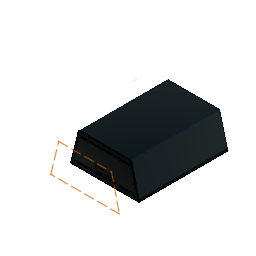
Assembly 4 v6 (Autodesk Fusion 360 archive; units mm, degrees)
design "Container_LeftBack"
Autodesk Fusion 360 part; units mm, degrees
sketch "Sketch1" plane through (0, 0, 0) normal (0, 1, 0) x (1, 0, 0)
  line L0 (-40, 14) -> (125, 14)
  line L1 (-20.5, -60) -> (105.5, -60)
  line L2 (-20.5, -60) -> (-40, 14)
  line L3 (105.5, -60) -> (125, 14)
  line L4 (-45.1906, 18) -> (130.1906, 18)
  line L5 (108.5825, -64) -> (130.1906, 18)
  line L6 (-23.5825, -64) -> (108.5825, -64)
  line L7 (-23.5825, -64) -> (-45.1906, 18)
  dimension "d6" = 4
  constraint horizontal L0
  constraint parallel L0 L1
extrude "Extrude1" add sketch "Sketch1" along normal blind 228
sketch "Sketch2" plane through (0, 0, 0) normal (0, 1, 0) x (1, 0, 0)
  line L0 (-45.3287, 17.7134) -> (130, 17.7134)
  line L1 (-25, -65) -> (110, -65)
  line L2 (110, -65) -> (130, 17.7134)
  line L3 (-25, -65) -> (-45.3287, 17.7134)
  constraint horizontal L0
  constraint horizontal L1
extrude "Extrude2" add sketch "Sketch2" along normal blind 1
sketch "Sketch3" plane through (0, 0, 0) normal (0, 1, 0) x (1, 0, 0)
  line L0 (20, 0) -> (65, 0)
  line L1 (65, 0) -> (65, -8.5)
  line L2 (65, -8.5) -> (20, -8.5)
  line L3 (20, -8.5) -> (20, 0)
  dimension "d12" = 8.5
  constraint horizontal L0
  constraint vertical L1
  constraint horizontal L2
  constraint vertical L3
  measures "d12" distance of L0.start L2.end
extrude "Extrude3" cut sketch "Sketch3" along normal blind 5
sketch "Sketch4" plane through (0, 0, 0) normal (0, 1, 0) x (1, 0, 0)
sketch "Sketch5" plane through (0, 0, 64) normal (0, 0, 1) x (-1, 0, 0)
  line L0 (23.5825, -1) -> (-108.5825, -1)
  line L1 (-108.5825, -1) -> (-108.5825, -228)
  line L2 (-108.5825, -228) -> (23.5825, -228)
  line L3 (23.5825, -228) -> (23.5825, -1)
sketch "Sketch6" plane through (0, 0, 0) normal (0, 1, 0) x (1, 0, 0)
split_face "SplitFace1" 2 faces at (20.4725, 76.6667, 64) (122.4972, 152.3333, 11.1953) by plane through (0, 0, 0) normal (0, -1, 0)
sketch "Sketch7" plane through (0, 0, 0) normal (0, 1, 0) x (1, 0, 0)
  line L0 (-25, -65, -50) -> (110, -65, -50) construction
  line L1 (110, -65, -50) -> (130.0131, 17.8851, -50) construction
  line L2 (130.0131, 17.8851, -50) -> (-45.0122, 17.8851, -50) construction
  line L3 (-45.0122, 17.8851, -50) -> (-25, -65, -50) construction
sketch "Sketch8" plane through (117.302, 0, 30.9107) normal (0.96699, 0, 0.254815) x (0, 1, 0)
  line L0 (1, -44.8037) -> (228, -44.8037)
  line L1 (228, -44.8037) -> (228, 34.2189)
  line L2 (228, 34.2189) -> (1, 34.2189)
  line L3 (1, 34.2189) -> (1, -44.8037)
sketch "Sketch9" plane through (0, 0, 0) normal (1, 0, 0) x (0, 1, 0)
sketch "Sketch10" plane through (0, 1, 0) normal (0, 1, 0) x (-1, 0, 0)
  line L0 (-20, 8.5) -> (-20, 0)
  line L1 (-20, 0) -> (-65, 0)
  line L2 (-65, 0) -> (-65, 8.5)
  line L3 (-65, 8.5) -> (-20, 8.5)
  line L4 (-105.5, 60) -> (-125, -14)
  line L5 (-125, -14) -> (40, -14)
  line L6 (40, -14) -> (20.5, 60)
  line L7 (20.5, 60) -> (-105.5, 60)
sketch "Sketch11" plane through (0, 1, 0) normal (0, 1, 0) x (-1, 0, 0)
  line L0 (-110, 55) -> (26.2971, 55)
  line L1 (26.2971, 55) -> (26.2971, 51.5)
  line L2 (26.2971, 51.5) -> (-110, 51.5)
  line L3 (-110, 51.5) -> (-110, 55)
  dimension "d16" = 3.5
  constraint horizontal L0
  constraint vertical L1
  constraint horizontal L2
  constraint vertical L3
  measures "d16" distance of L0.start L2.end
extrude "Extrude4" add sketch "Sketch11" along normal blind 227
sketch "Sketch12" plane through (0, 1, 0) normal (0, 1, 0) x (-1, 0, 0)
  line L0 (-124.605, -9) -> (40, -9)
  line L1 (40, -9) -> (40, -5.5)
  line L2 (40, -5.5) -> (-124.605, -5.5)
  line L3 (-124.605, -5.5) -> (-124.605, -9)
  dimension "d19" = 3.5
  constraint horizontal L0
  constraint vertical L1
  constraint horizontal L2
  constraint vertical L3
  measures "d19" distance of L0.start L2.end
extrude "Extrude5" add sketch "Sketch12" along normal blind 227
sketch "Sketch13" plane through (-152.3278, -0.2738, -0.1145) normal (-0.999998, -0.001797, -0.000752) x (0.001797, -0.999998, 0)
  line L0 (-277.193, -23.2673) -> (-277.1579, -25.267)
  line L1 (-277.1579, -25.267) -> (-275.1582, -25.2318)
  line L2 (-275.1582, -25.2318) -> (-262.1602, -25.0033)
  line L3 (-262.1602, -25.0033) -> (-262.1953, -23.0037)
  line L4 (-262.1953, -23.0037) -> (-277.193, -23.2673)
sketch "Sketch14" plane through (0, 228, 0) normal (0, 1, 0) x (-1, 0, 0)
  line L0 (-122.7601, -5.5) -> (-107.7399, 51.5)
  line L1 (-107.7399, 51.5) -> (22.7399, 51.5)
  line L2 (22.7399, 51.5) -> (37.7601, -5.5)
  line L3 (37.7601, -5.5) -> (-122.7601, -5.5)
  line L4 (-123.6824, -9) -> (38.6824, -9)
  line L5 (38.6824, -9) -> (40, -14)
  line L6 (40, -14) -> (-125, -14)
  line L7 (-125, -14) -> (-123.6824, -9)
  line L8 (-106.8176, 55) -> (-105.5, 60)
  line L9 (-105.5, 60) -> (20.5, 60)
  line L10 (20.5, 60) -> (21.8176, 55)
  line L11 (21.8176, 55) -> (-106.8176, 55)
  line L12 (25.9541, 55) -> (23.5825, 64)
  line L13 (23.5825, 64) -> (-108.5825, 64)
  line L14 (-108.5825, 64) -> (-128.7186, -12.414)
  line L15 (-128.7186, -12.414) -> (-130.1906, -18)
  line L16 (-130.1906, -18) -> (45.1906, -18)
  line L17 (45.1906, -18) -> (26.2971, 53.6986)
  line L18 (26.2971, 53.6986) -> (26.2971, 55)
  line L19 (26.2971, 55) -> (25.9541, 55)
  line L20 (20.5, 60) -> (26.2487, 60)
  line L21 (26.2487, 60) -> (27.5, 55)
  line L22 (27.5, 55) -> (21.8176, 55)
  line L23 (20.5, 60) -> (21.8176, 55)
  constraint coincident L9.end L10.start
  constraint parallel L9 L20
  constraint coincident L10.end L11.start
extrude "Extrude6" cut sketch "Sketch14" against normal blind 16 contours L10 L12 L20 L22 L23 | L12 L19 L20 L21 L22
sketch "Sketch15" plane through (0, 228, 0) normal (0, 1, 0) x (-1, 0, 0)
  line L0 (25.9541, 55) -> (21.8176, 55)
  line L1 (21.8176, 55) -> (-106.8176, 55)
  line L2 (-106.8176, 55) -> (-105.5, 60)
  line L3 (-105.5, 60) -> (24.6365, 60)
  line L4 (24.6365, 60) -> (23.5825, 64)
  line L5 (23.5825, 64) -> (-108.5825, 64)
  line L6 (-108.5825, 64) -> (-128.7186, -12.414)
  line L7 (-128.7186, -12.414) -> (-130.1906, -18)
  line L8 (-130.1906, -18) -> (45.1906, -18)
  line L9 (45.1906, -18) -> (26.2971, 53.6986)
  line L10 (26.2971, 53.6986) -> (26.2971, 55)
  line L11 (26.2971, 55) -> (25.9541, 55)
  line L12 (-122.7601, -5.5) -> (-107.7399, 51.5)
  line L13 (-107.7399, 51.5) -> (22.7399, 51.5)
  line L14 (22.7399, 51.5) -> (37.7601, -5.5)
  line L15 (37.7601, -5.5) -> (-122.7601, -5.5)
  line L16 (-123.6824, -9) -> (38.6824, -9)
  line L17 (38.6824, -9) -> (40, -14)
  line L18 (40, -14) -> (-125, -14)
  line L19 (-125, -14) -> (-123.6824, -9)
  line L20 (38.6824, -9) -> (43.5, -9)
  line L21 (43.5, -9) -> (44.5, -14)
  line L22 (44.5, -14) -> (40, -14)
  line L23 (38.6824, -9) -> (40, -14)
  dimension "d25" = 0
  constraint coincident L16.end L17.start
  constraint parallel L16 L20
  constraint coincident L17.end L18.start
extrude "Extrude7" cut sketch "Sketch15" against normal blind 16 contours L9 L20 L21 L22 | L9 L17 L20 L22 L23

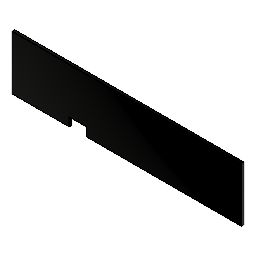
design "LC_SFPB: Left Side (Front to Back"
Autodesk Fusion 360 part; units mm, degrees
sketch "Sketch1" plane through (0, 0, 0) normal (0, 1, 0) x (1, 0, 0)
  line L0 (-110, -30) -> (290, -30)
  line L1 (290, -30) -> (290, 65)
  line L2 (290, 65) -> (-110, 65)
  line L3 (-110, 65) -> (-110, -30)
  line L4 (290, 65) -> (20, 65)
  line L5 (20, 65) -> (20, 50)
  line L6 (20, 50) -> (-10, 50)
  line L7 (-10, 50) -> (-10, 65)
  constraint horizontal L0
  constraint perpendicular L0 L1
  constraint perpendicular L1 L2
  constraint perpendicular L0 L3
  constraint coincident L2 L4.end
  constraint perpendicular L2 L5
  constraint perpendicular L5 L6
  constraint coincident L2 L7.end
  constraint perpendicular L2 L7
extrude "Extrude1" add sketch "Sketch1" along normal blind 5 contours L0 L1 L2 L3 L4 L5 L6 L7
sketch "Sketch2" plane through (0, 0, 0) normal (0, 1, 0) x (1, 0, 0)

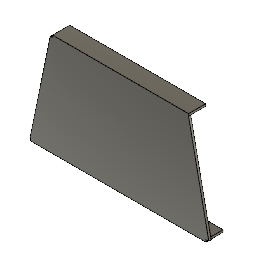
design "Door (Height needs adjustment maybe)"
Autodesk Fusion 360 part; units mm, degrees
sketch "Sketch1" plane through (0, 0, 0) normal (0, 1, 0) x (1, 0, 0)
  line L0 (-30, -40) -> (90, -40)
  line L1 (90, 45) -> (-30, 45)
  line L2 (-30, 45) -> (-47.5, 45)
  line L3 (90, 45) -> (107.5, 45)
  line L4 (-47.5, 45) -> (-30, -40)
  line L5 (107.5, 45) -> (90, -40)
  constraint horizontal L0
extrude "Extrude1" add sketch "Sketch1" along normal blind 2
sketch "Sketch2" plane through (0, 0, 0) normal (1, 0, 0) x (0, 1, 0)
  line L0 (0, 40) -> (15, 40)
  line L1 (15, 40) -> (15, 42)
  line L2 (15, 42) -> (0, 42)
  line L3 (0, 42) -> (0, 40)
  line L4 (0, -45) -> (0, -47)
  line L5 (0, -47) -> (15, -47)
  line L6 (15, -47) -> (15, -45)
  line L7 (15, -45) -> (0, -45)
  constraint horizontal L0
  constraint perpendicular L0 L1
  constraint perpendicular L1 L2
  constraint perpendicular L0 L3
  constraint vertical L4
  constraint perpendicular L4 L5
  constraint perpendicular L5 L6
  constraint perpendicular L4 L7
extrude "Extrude2" add sketch "Sketch2" along normal blind 105 and the other way blind 47 contours L4 L5 L6 L7
sketch "Sketch3" plane through (0, 0, 0) normal (1, 0, 0) x (0, 1, 0)
  line L0 (0, 40) -> (15, 40)
  line L1 (15, 40) -> (15, 42)
  line L2 (15, 42) -> (0, 42)
  line L3 (0, 42) -> (0, 40)
  constraint horizontal L0
  constraint perpendicular L0 L1
  constraint perpendicular L1 L2
  constraint perpendicular L0 L3
extrude "Extrude3" add sketch "Sketch3" along normal blind 90 and the other way blind 28

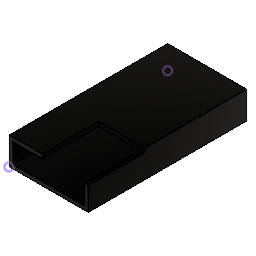
design "Left Pavement"
Autodesk Fusion 360 part; units mm, degrees
sketch "Sketch1" plane through (0, 0, 0) normal (0, 1, 0) x (1, 0, 0)
  line L0 (-30, 0) -> (70, 0)
  line L1 (70, 0) -> (70, -35)
  line L2 (70, -35) -> (-30, -35)
  line L3 (-30, -35) -> (-30, 0)
  line L4 (-25, -5) -> (65, -5)
  line L5 (65, -5) -> (65, -30)
  line L6 (65, -30) -> (-25, -30)
  line L7 (-25, -30) -> (-25, -5)
  dimension "d1" = 35
  dimension "d2" = 5
  constraint horizontal L0
  constraint perpendicular L0 L1
  constraint perpendicular L1 L2
  constraint perpendicular L0 L3
  measures "d1" distance of L0.end L1.end
extrude "Extrude1" add sketch "Sketch1" along normal blind 200 makes body 1
sketch "Sketch2" plane through (70, 0, 0) normal (1, 0, 0) x (0, 1, 0)
  line L0 (0, 35) -> (0, 0)
  line L1 (0, 0) -> (200, 0)
  line L2 (200, 0) -> (200, 35)
  line L3 (200, 35) -> (0, 35)
  line L4 (200, 0) -> (360, 0)
  line L5 (360, 0) -> (360, 5)
  line L6 (360, 5) -> (200, 5)
  line L7 (200, 0) -> (200, 5)
  constraint coincident L1.end L2.start
  constraint perpendicular L2 L4
  constraint perpendicular L4 L5
  constraint coincident L2 L6.end
  constraint perpendicular L2 L6
extrude "Extrude2" add sketch "Sketch2" against normal blind 100 contours L2 L4 L5 L6 L7 bodies 1
sketch "Sketch3" plane through (0, 0, 0) normal (1, 0, 0) x (0, 1, 0)
sketch "Sketch4" plane through (-30, 0, 0) normal (-1, 0, 0) x (0, -1, 0)
  line L0 (0, 0) -> (0, 35)
  line L1 (0, 35) -> (-200, 35)
  line L2 (-200, 35) -> (-200, 5)
  line L3 (-360, 5) -> (-360, 0)
sketch "Sketch5" plane through (0, 0, 0) normal (0, 1, 0) x (1, 0, 0)
split_face "SplitFace1" 2 faces at (5, 306.6667, 5) (36.6667, 66.6667, 35) by plane through (70, 0, 0) normal (1, 0, 0) on bodies 1
sketch "Sketch6" plane through (0, 0, 5) normal (0, 0, 1) x (-1, 0, 0)
  line L0 (25, 0) -> (-65, 0)
  line L1 (-65, 0) -> (-65, -200)
  line L2 (-65, -200) -> (-70, -200)
  line L3 (-70, -200) -> (-70, -360)
  line L4 (-70, -360) -> (30, -360)
  line L5 (30, -360) -> (30, -200)
  line L6 (30, -200) -> (25, -200)
  line L7 (25, -200) -> (25, 0)
  line L8 (30, -200) -> (-70, -200)
  line L9 (-70, -200) -> (-70, -207.0098)
  line L10 (-70, -207.0098) -> (30, -207.0098)
  line L11 (30, -207.0098) -> (30, -200)
  constraint horizontal L8
  constraint vertical L9
  constraint horizontal L10
  constraint vertical L11
  constraint coincident L3 L9.end
  constraint coincident L5.end L6.start
extrude "Extrude3" cut sketch "Sketch6" against normal blind 25 contours L2 L3 L5 L6 L8 L9 L10 L11 bodies 1 makes body 2 at (3.3333, 309.0033, 0)
sketch "Sketch7" plane through (0, 0, 35) normal (0, 0, 1) x (-1, 0, 0)
  line L0 (30, 0) -> (-70, 0)
  line L1 (-70, 0) -> (-70, -200)
  line L2 (-70, -200) -> (30, -200)
  line L3 (30, -200) -> (30, 0)
  line L4 (-70, 0) -> (-12, 0)
  line L5 (-12, 0) -> (-12, -71)
  line L6 (-12, -71) -> (-70, -71)
  line L7 (-70, -71) -> (-70, 0)
  dimension "d10" = 58
  dimension "d11" = 71
  constraint coincident L0.end L1.start
  constraint perpendicular L1 L4
  constraint perpendicular L0 L5
  constraint coincident L1 L6.end
  constraint perpendicular L1 L6
  measures "d10" distance of L0.end L4.end
  measures "d11" distance of L4.end L5.end
extrude "Extrude4" cut sketch "Sketch7" against normal blind 5 contours L0 L1 L4 L5 L6 L7 bodies 1
hidden bodies 2

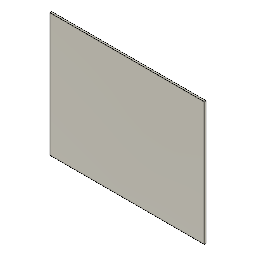
design "LC_SFPB: Floor"
Autodesk Fusion 360 part; units mm, degrees
sketch "Sketch1" plane through (0, 0, 0) normal (0, 1, 0) x (1, 0, 0)
  line L0 (-375, 0) -> (125, 0)
  line L1 (125, 0) -> (125, 400)
  line L2 (125, 400) -> (-375, 400)
  line L3 (-375, 400) -> (-375, 0)
  dimension "d1" = 500
  constraint horizontal L0
  constraint perpendicular L0 L1
  constraint perpendicular L1 L2
  constraint perpendicular L0 L3
  measures "d1" distance of L1.end L2.end
extrude "Extrude1" add sketch "Sketch1" along normal blind 6
